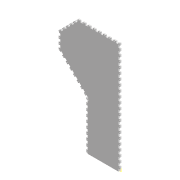
# Autodesk Inventor part: 00_Baseplate_Simmo_base
Saved by Autodesk Inventor 2022 (Build 260153000, 153)
## iProperties
Created: 2022-04-28
Part Number: 00_Baseplate_Simmo_base
Material: Generisch
Document SubType Name: Modeling
Designer: diederichbenedict
Density: 1 g/cm^3
Appearance: Vorgabe
Author: diederichbenedict
Autodesk Inventor part; units mm, degrees
ref_plane "YZ Plane" through (0, 0, 0) normal (1, 0, 0) x (0, 1, 0)
ref_plane "XZ Plane" through (0, 0, 0) normal (0, 1, 0) x (-1, 0, 0)
ref_plane "XY Plane" through (0, 0, 0) normal (0, 0, 1) x (1, 0, 0)
ref_plane "Arbeitsebene1" through (0, 0, 0) normal (0, 0, 1) x (1, 0, 0)
sketch "Skizze1" plane through (0, 0, 0) normal (0, 0, 1) x (1, 0, 0)
  line L0 (91.8818, 443.0401) -> (90.2278, 433.6598) projected
  line L1 (120, 0) -> (126, 0)
  line L2 (126, 0) -> (126, 438)
  line L3 (126, 438) -> (-39, 438)
  line L4 (-39, 438) -> (-114, 363)
  line L5 (-114, 363) -> (-114, 298)
  line L6 (-114, 298) -> (-6, 190)
  line L7 (-6, 190) -> (-6, 0)
  circle A0 centre (58.4, 5) radius 2.95 projected
  line L8 (120, 0) -> (0, 0) projected
  line L9 (0, 0) -> (0, 10) projected
  line L10 (120, 10) -> (0, 10) projected
  line L11 (120, 0) -> (120, 10) projected
  line L12 (120, 0) -> (0, 0)
  line L13 (126, 0) -> (-6, 0)
  point P0 (126, 5)
  dimension "d0" = 135
  dimension "d1" = 135
  dimension "d2" = 165
  dimension "d4" = 75
  dimension "d5" = 65
  dimension "d66" = 190
  dimension "d67" = 6
  dimension "d68" = 6
  constraints: 18 end point, 3 horizontal, 2 perpendicular, 1 parallel, 1 point on line
  measures "d0" angle of L7 L6
  measures "d1" angle of L5 L4
  measures "d2" distance from line of L2 L3.end
  measures "d4" horizontal distance of L4.end L3.end
  measures "d5" distance of L4.end L5.end
  measures "d66" vertical distance of L1.start L6.end
  measures "d67" distance between parallel lines of L11 L2
  measures "d68" distance between parallel lines of L7 L9
extrude "Extrusion1" add sketch "Skizze1" along normal blind 5 contours L11 L10 L9 L13 L7 L6 L5 L4 L3 L2 L1 | L8 L9 L10 L11 | A0
sketch "Skizze2" plane through (0, 0, 0) normal (0, 0, -1) x (-1, 0, 0)
  line L0 (-126, 0) -> (-120, 0)
  line L1 (-120, 0) -> (-120, 10)
  line L2 (-120, 10) -> (-126, 10)
  line L3 (-126, 10) -> (-126, 0)
  circle A0 centre (-123, 15) radius 1.5
  point P0 (0, 0)
  dimension "d8" = 6
  dimension "d9" = 10
  dimension "d15" = 3
  dimension "d16" = 5
  constraints: 8 end point, 2 parallel, 2 point on line, 1 centre point, 1 horizontal, 1 perpendicular
  measures "d8" distance of L2.end L1.end
  measures "d9" distance of L1.end L0.end
  measures "d15" diameter of A0
  measures "d16" distance from line of A0.centre L2
extrude "Extrusion2" cut sketch "Skizze2" against normal through all
sketch "Skizze3" plane through (0, 0, 0) normal (0, 0, -1) x (-1, 0, 0)
  line L0 (114, 298) -> (6, 190) projected
  line L1 (114, 363) -> (114, 298) projected
  line L2 (39, 438) -> (114, 363) projected
  line L3 (-126, 438) -> (39, 438) projected
  line L4 (-120, 10) -> (-120, 438) projected
  line L5 (0, 190) -> (0, 0) projected
pattern_linear "Rechteckige Anordnung1" count 24 spacing 20 along (0, 1, 0) of "Extrusion2"
sketch "Skizze4" plane through (0, 0, 0) normal (0, 0, -1) x (-1, 0, 0)
  line L0 (-120, 438) -> (-110, 438)
  line L1 (-110, 438) -> (-110, 432)
  line L2 (-110, 432) -> (-120, 432)
  line L3 (-120, 432) -> (-120, 438)
  circle A0 centre (-105, 435) radius 1.5
  line L4 (-126, 438) -> (39, 438) projected
  line L5 (-120, 0) -> (-120, 450) projected
  point P0 (0, 0)
  dimension "d17" = 10
  dimension "d18" = 6
  dimension "d19" = 3
  dimension "d20" = 5
  constraints: 8 end point, 2 parallel, 2 point on line, 1 centre point, 1 horizontal, 1 perpendicular
  measures "d17" distance of L1.end L2.end
  measures "d18" distance of L0.end L1.end
  measures "d19" diameter of A0
  measures "d20" distance from line of A0.centre L1
extrude "Extrusion3" cut sketch "Skizze4" against normal through all
pattern_linear "Rechteckige Anordnung2" count 24 spacing 20 along (-1, 0, 0) of "Extrusion3"
sketch "Skizze5" plane through (0, 0, 0) normal (0, 0, -1) x (-1, 0, 0)
  line L0 (39, 438) -> (40, 437) projected
  line L1 (30, 438) -> (39, 438) projected
  line L2 (6, 190) -> (6, 0) projected
  line L3 (114, 298) -> (6, 190) projected
  line L4 (114, 363) -> (114, 298) projected
  line L5 (45, 432) -> (40.7574, 427.7574)
  line L6 (40.7574, 427.7574) -> (47.8284, 420.6863)
  line L7 (47.8284, 420.6863) -> (52.0711, 424.9289)
  line L8 (52.0711, 424.9289) -> (45, 432)
  circle A0 centre (53.4853, 419.2721) radius 1.5
  line L9 (6, 0) -> (-120, 0) projected
  line L10 (-126, 10) -> (-126, 20) projected
  line L11 (-120, 10) -> (-120, 0) projected
  line L12 (-126, 10) -> (-120, 10) projected
  line L13 (-120, 420) -> (-126, 420) projected
  line L14 (-126, 410) -> (-126, 420) projected
  line L15 (-126, 410) -> (-120, 410) projected
  line L16 (-120, 410) -> (-120, 400) projected
  line L17 (-120, 400) -> (-126, 400) projected
  line L18 (-126, 390) -> (-126, 400) projected
  line L19 (-126, 390) -> (-120, 390) projected
  line L20 (-120, 390) -> (-120, 380) projected
  line L21 (-120, 380) -> (-126, 380) projected
  line L22 (-126, 370) -> (-126, 380) projected
  line L23 (-126, 370) -> (-120, 370) projected
  line L24 (-120, 370) -> (-120, 360) projected
  line L25 (-120, 360) -> (-126, 360) projected
  line L26 (-126, 350) -> (-126, 360) projected
  line L27 (-126, 350) -> (-120, 350) projected
  line L28 (-120, 350) -> (-120, 340) projected
  line L29 (-120, 340) -> (-126, 340) projected
  line L30 (-126, 330) -> (-126, 340) projected
  line L31 (-126, 330) -> (-120, 330) projected
  line L32 (-120, 330) -> (-120, 320) projected
  line L33 (-120, 320) -> (-126, 320) projected
  line L34 (-126, 310) -> (-126, 320) projected
  line L35 (-126, 310) -> (-120, 310) projected
  line L36 (-120, 310) -> (-120, 300) projected
  line L37 (-120, 300) -> (-126, 300) projected
  line L38 (-126, 290) -> (-126, 300) projected
  line L39 (-126, 290) -> (-120, 290) projected
  line L40 (-120, 290) -> (-120, 280) projected
  line L41 (-120, 280) -> (-126, 280) projected
  line L42 (-126, 270) -> (-126, 280) projected
  line L43 (-126, 270) -> (-120, 270) projected
  line L44 (-120, 270) -> (-120, 260) projected
  line L45 (-120, 260) -> (-126, 260) projected
  line L46 (-126, 250) -> (-126, 260) projected
  line L47 (-126, 250) -> (-120, 250) projected
  line L48 (-120, 250) -> (-120, 240) projected
  line L49 (-120, 240) -> (-126, 240) projected
  line L50 (-126, 230) -> (-126, 240) projected
  line L51 (-126, 230) -> (-120, 230) projected
  line L52 (-120, 230) -> (-120, 220) projected
  line L53 (-120, 220) -> (-126, 220) projected
  line L54 (-126, 210) -> (-126, 220) projected
  line L55 (-126, 210) -> (-120, 210) projected
  line L56 (-120, 210) -> (-120, 200) projected
  line L57 (-120, 200) -> (-126, 200) projected
  line L58 (-126, 190) -> (-126, 200) projected
  line L59 (-126, 190) -> (-120, 190) projected
  line L60 (-120, 190) -> (-120, 180) projected
  line L61 (-120, 180) -> (-126, 180) projected
  line L62 (-126, 170) -> (-126, 180) projected
  line L63 (-126, 170) -> (-120, 170) projected
  line L64 (-120, 170) -> (-120, 160) projected
  line L65 (-120, 160) -> (-126, 160) projected
  line L66 (-126, 150) -> (-126, 160) projected
  line L67 (-126, 150) -> (-120, 150) projected
  line L68 (-120, 150) -> (-120, 140) projected
  line L69 (-120, 140) -> (-126, 140) projected
  line L70 (-126, 130) -> (-126, 140) projected
  line L71 (-126, 130) -> (-120, 130) projected
  line L72 (-120, 130) -> (-120, 120) projected
  line L73 (-120, 120) -> (-126, 120) projected
  line L74 (-126, 110) -> (-126, 120) projected
  line L75 (-126, 110) -> (-120, 110) projected
  line L76 (-120, 110) -> (-120, 100) projected
  line L77 (-120, 100) -> (-126, 100) projected
  line L78 (-126, 90) -> (-126, 100) projected
  line L79 (-126, 90) -> (-120, 90) projected
  line L80 (-120, 90) -> (-120, 80) projected
  line L81 (-120, 80) -> (-126, 80) projected
  line L82 (-126, 70) -> (-126, 80) projected
  line L83 (-126, 70) -> (-120, 70) projected
  line L84 (-120, 70) -> (-120, 60) projected
  line L85 (-120, 60) -> (-126, 60) projected
  line L86 (-126, 50) -> (-126, 60) projected
  line L87 (-126, 50) -> (-120, 50) projected
  line L88 (-120, 50) -> (-120, 40) projected
  line L89 (-120, 40) -> (-126, 40) projected
  line L90 (-126, 30) -> (-126, 40) projected
  line L91 (-126, 30) -> (-120, 30) projected
  line L92 (-120, 30) -> (-120, 20) projected
  line L93 (-120, 20) -> (-126, 20) projected
  line L94 (-126, 430) -> (-126, 438) projected
  line L95 (-126, 430) -> (-120, 430) projected
  line L96 (-120, 430) -> (-120, 420) projected
  line L97 (40, 432) -> (40, 437) projected
  line L98 (30, 438) -> (30, 432) projected
  line L99 (30, 432) -> (20, 432) projected
  line L100 (20, 432) -> (20, 438) projected
  line L101 (10, 438) -> (20, 438) projected
  line L102 (10, 438) -> (10, 432) projected
  line L103 (10, 432) -> (0, 432) projected
  line L104 (0, 432) -> (0, 438) projected
  line L105 (-10, 438) -> (0, 438) projected
  line L106 (-10, 438) -> (-10, 432) projected
  line L107 (-10, 432) -> (-20, 432) projected
  line L108 (-20, 432) -> (-20, 438) projected
  line L109 (-30, 438) -> (-20, 438) projected
  line L110 (-30, 438) -> (-30, 432) projected
  line L111 (-30, 432) -> (-40, 432) projected
  line L112 (-40, 432) -> (-40, 438) projected
  line L113 (-50, 438) -> (-40, 438) projected
  line L114 (-50, 438) -> (-50, 432) projected
  line L115 (-50, 432) -> (-60, 432) projected
  line L116 (-60, 432) -> (-60, 438) projected
  line L117 (-70, 438) -> (-60, 438) projected
  line L118 (-70, 438) -> (-70, 432) projected
  line L119 (-70, 432) -> (-80, 432) projected
  line L120 (-80, 432) -> (-80, 438) projected
  line L121 (-90, 438) -> (-80, 438) projected
  line L122 (-90, 438) -> (-90, 432) projected
  line L123 (-90, 432) -> (-100, 432) projected
  line L124 (-100, 432) -> (-100, 438) projected
  line L125 (-110, 438) -> (-100, 438) projected
  line L126 (-110, 438) -> (-110, 432) projected
  line L127 (-110, 432) -> (-120, 432) projected
  line L128 (-120, 432) -> (-120, 438) projected
  line L129 (-126, 438) -> (-120, 438) projected
  line L130 (45, 432) -> (114, 363) projected
  line L131 (45, 432) -> (40, 432) projected
  line L132 (45, 432) -> (114, 363) projected
  point P0 (0, 0)
  dimension "d29" = 6
  dimension "d30" = 10
  dimension "d31" = 3
  dimension "d32" = 5
  constraints: 8 end point, 3 parallel, 1 centre point, 1 perpendicular
  measures "d29" distance of L5.start L5.end
  measures "d30" distance of L6.end L5.end
  measures "d31" diameter of A0
  measures "d32" distance from line of A0.centre L7
extrude "Extrusion4" cut sketch "Skizze5" against normal through all contours L8 L7 L6 L5 | A0
pattern_linear "Rechteckige Anordnung3" count 24 spacing 20 along (-0.7071068, -0.7071068, 0) of "Extrusion4"
sketch "Skizze6" plane through (0, 0, 0) normal (0, 0, -1) x (-1, 0, 0)
  line L0 (114, 363) -> (114, 298) projected
  line L1 (114, 354.5147) -> (108, 354.5147)
  line L2 (108, 354.5147) -> (108, 344.5147)
  line L3 (108, 344.5147) -> (114, 344.5147)
  line L4 (114, 344.5147) -> (114, 354.5147)
  circle A0 centre (111, 339.5147) radius 1.5
  point P0 (0, 0)
  point P1 (114, 344.5147)
  point P2 (114, 356.5147)
  dimension "d38" = 6
  dimension "d39" = 10
  dimension "d40" = 3
  dimension "d41" = 5
  constraints: 6 end point, 2 horizontal, 1 centre point, 1 parallel, 1 vertical, 3 other
  measures "d38" distance of L1.start L1.end
  measures "d39" distance of L3.start L1.end
  measures "d40" diameter of A0
  measures "d41" distance from line of A0.centre L3
extrude "Extrusion5" cut sketch "Skizze6" against normal through all
pattern_linear "Rechteckige Anordnung4" count 24 spacing 20 along (0, -1, 0) of "Extrusion5"
sketch "Skizze7" plane through (0, 0, 0) normal (0, 0, -1) x (-1, 0, 0)
  line L0 (114, 298) -> (6, 190) projected
  line L1 (114, 298) -> (6, 190) projected
  line L2 (108, 292) -> (103.7574, 296.2426)
  line L3 (103.7574, 296.2426) -> (96.6863, 289.1716)
  line L4 (96.6863, 289.1716) -> (100.9289, 284.9289)
  line L5 (100.9289, 284.9289) -> (108, 292)
  line L6 (108, 292) -> (114, 292) construction
  circle A0 centre (95.2721, 283.5147) radius 1.5
  point P0 (0, 0)
  dimension "d47" = 6
  dimension "d48" = 135
  dimension "d49" = 10
  dimension "d50" = 3
  dimension "d51" = 5
  constraints: 10 end point, 2 parallel, 2 perpendicular, 1 centre point, 1 equal length, 1 horizontal
  measures "d47" distance of L2.start L2.end
  measures "d48" angle of L6 L2
  measures "d49" distance of L3.end L2.end
  measures "d50" diameter of A0
  measures "d51" distance from line of L4 A0.centre
extrude "Extrusion6" cut sketch "Skizze7" against normal through all
pattern_linear "Rechteckige Anordnung5" count 8 spacing 20 along (0.7071068, -0.7071068, 0) of "Extrusion6"
sketch "Skizze8" plane through (0, 0, 0) normal (0, 0, -1) x (-1, 0, 0)
  line L0 (0, 183.2478) -> (0, 173.2478)
  line L1 (0, 173.2478) -> (5.4242, 173.2478)
  circle A0 centre (3, 168.2478) radius 1.5
  line L2 (6, 190) -> (6, 0) projected
  line L3 (0, 173.2478) -> (6, 173.2478)
  line L4 (6, 173.2478) -> (6, 183.2478)
  line L5 (6, 183.2478) -> (0, 183.2478)
  line L6 (0, 183.2478) -> (0, 173.2478)
  dimension "d58" = 10
  dimension "d59" = 3
  dimension "d60" = 5
  constraints: 12 end point, 2 parallel, 1 centre point, 1 horizontal, 1 perpendicular, 1 point on line
  measures "d58" distance of L0.end L0.start
  measures "d59" diameter of A0
  measures "d60" distance from line of A0.centre L1
extrude "Extrusion7" cut sketch "Skizze8" against normal through all
pattern_linear "Rechteckige Anordnung6" count 24 spacing 20 along (0, -1, 0) of "Extrusion7"
equation "\"d16\" = 0.5 * d9"
equation "\"d17\" = d9"
equation "\"d20\" = 0.5 * d9"
equation "\"d30\" = d9"
equation "\"d32\" = 0.5 * d9"
equation "\"d39\" = d9"
equation "\"d41\" = 0.5 * d9"
equation "\"d49\" = d9"
equation "\"d51\" = 0.5 * d9"
equation "\"d56\" = 2 * d9"
equation "\"d60\" = 0.5 * d9"
equation "\"d14\" = 2 * d9"
equation "\"d25\" = 2 * d9"
equation "\"d37\" = 2 * d9"
equation "\"d46\" = 2 * d9"
equation "\"d65\" = 2 * d9"
